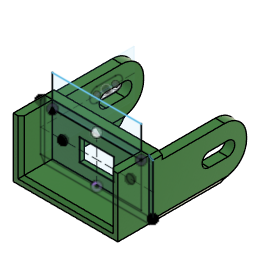
Sensorhalter v8 (Autodesk Fusion 360 design; units mm, degrees)
Autodesk Fusion 360 part; units mm, degrees
sketch "Skizze1" plane through (0, 0, 0) normal (0, 0, 1) x (1, 0, 0)
  line L0 (-18, 30) -> (-18, 0)
  line L1 (-18, 0) -> (18, 0)
  line L2 (18, 0) -> (18, 30)
  line L3 (18, 30) -> (15, 30)
  line L4 (15, 30) -> (15, 3)
  line L5 (15, 3) -> (-15, 3)
  line L6 (-15, 3) -> (-15, 30)
  line L7 (-15, 30) -> (-18, 30)
  line L8 (0, 75) -> (0, -25) construction
  dimension "d1" = 3
  dimension "d2" = 3
  dimension "d3" = 36
  dimension "d4" = 30
  constraint vertical L0
  constraint perpendicular L0 L1
  constraint perpendicular L1 L2
  constraint perpendicular L2 L3
  constraint perpendicular L3 L4
  constraint perpendicular L4 L5
  constraint perpendicular L5 L6
  constraint perpendicular L0 L7
  constraint perpendicular L1 L8
  constraint symmetric L0 L2 L8
  constraint equal L0 L2
  measures "d1" distance of L6.end L0.start
  measures "d2" distance of L1 L5
  measures "d3" distance of L0 L2
  measures "d4" distance of L1 L7
extrude "Extrusion1" add sketch "Skizze1" along normal blind 15
sketch "Skizze2" plane through (-18, 0, 0) normal (-1, 0, 0) x (0, -1, 0)
  line L0 (-30, 0) -> (0, 0)
  line L1 (0, 0) -> (0, 15)
  line L2 (0, 15) -> (-30, 15)
  line L3 (-30, 15) -> (-30, 0)
  line L4 (-30, 7.5) -> (0, 7.5) construction
  line L5 (-24, 9.75) -> (-18, 9.75)
  line L6 (-18, 5.25) -> (-24, 5.25)
  arc A0 (-24, 9.75) -> (-24, 5.25) centre (-24, 7.5) ccw
  arc A1 (-18, 5.25) -> (-18, 9.75) centre (-18, 7.5) ccw
  dimension "d7" = 4.5
  dimension "d8" = 6
  dimension "d9" = 6
  constraint midpoint L3 L4.start
  constraint midpoint L1 L4.end
  constraint coincident L4 A0.centre
  constraint coincident L4 A1.centre
  constraint equal A0 A1
  constraint tangent L5 A0
  constraint tangent L5 A1
  constraint tangent L6 A1
  constraint tangent L6 A0
  measures "d7" diameter of A0
  measures "d8" distance of L3 A0.centre
  measures "d9" distance of A0.centre A1.centre
extrude "Extrusion2" cut sketch "Skizze2" against normal up to surface (36 mm away) contours L5 L6 A0 A1
fillet "Abrundung1" radius 7 4 edges at (-16.5, 30, 15) (16.5, 30, 15) (16.5, 30, 0) (-16.5, 30, 0)
sketch "Skizze3" plane through (0, 0, 0) normal (0, -1, 0) x (1, 0, 0)
  line L0 (-18, 0) -> (18, 0)
  line L1 (18, 0) -> (18, 15)
  line L2 (18, 15) -> (-18, 15)
  line L3 (-18, 15) -> (-18, 0)
  line L4 (18, 7.5) -> (-18, 7.5) construction
  circle A0 centre (10.8, 7.5) radius 1.25
  circle A1 centre (-10.8, 7.5) radius 1.25
  line L5 (14.25, 0.5) -> (-14.25, 0.5)
  line L6 (-14.25, 0.5) -> (-14.25, 14.5)
  line L7 (-14.25, 14.5) -> (14.25, 14.5)
  line L8 (14.25, 14.5) -> (14.25, 0.5)
  line L9 (18, 0) -> (-18, 0)
  line L10 (-18, 0) -> (-18, 15)
  line L11 (18, 16.3062) -> (18, 0)
  line L12 (0, 0) -> (0, 15) construction
  line L13 (16.75, -2) -> (-16.75, -2)
  line L14 (-16.75, -2) -> (-16.75, 17)
  line L15 (-16.75, 17) -> (16.75, 17)
  line L16 (16.75, 17) -> (16.75, -2)
  line L17 (18, 0) -> (16.75, -2)
  line L18 (-18, 0) -> (-16.75, -2)
  line L19 (-18, 15) -> (-16.75, 17)
  line L20 (16.75, 17) -> (18, 16.3062)
  line L21 (-5.5, 4) -> (5.5, 4)
  line L22 (5.5, 4) -> (5.5, 11)
  line L23 (5.5, 11) -> (-5.5, 11)
  line L24 (-5.5, 11) -> (-5.5, 4)
  dimension "d14" = 2.5
  dimension "d15" = 21.6
  dimension "d16" = 14
  dimension "d17" = 28.5
  dimension "d18" = 2.5
  dimension "d19" = 2.5
  dimension "d20" = 2.5
  dimension "d21" = 2.5
  dimension "d28" = 11
  dimension "d29" = 7
  constraint midpoint L1 L4.start
  constraint midpoint L3 L4.end
  constraint coincident L4 A0.centre
  constraint coincident L4 A1.centre
  constraint horizontal L5
  constraint vertical L6
  constraint horizontal L7
  constraint vertical L8
  constraint horizontal L9
  constraint vertical L10
  constraint vertical L11
  constraint coincident L2.end L3.start
  constraint coincident L0.end L1.start
  constraint equal A0 A1
  constraint coincident L12.start origin
  constraint symmetric A0.centre A1.centre L12
  constraint symmetric L4 L5 L7
  constraint symmetric L6 L8 L12
  constraint horizontal L13
  constraint vertical L14
  constraint horizontal L15
  constraint vertical L16
  constraint horizontal L21
  constraint vertical L22
  constraint horizontal L23
  constraint vertical L24
  constraint symmetric L12 L22 L24
  constraint symmetric L4 L21 L23
  measures "d14" diameter of A0
  measures "d15" distance of A0.centre A1.centre
  measures "d16" distance of L5.end L6.end
  measures "d17" distance of L5.start L5.end
  measures "d18" distance of L8 L16
  measures "d19" distance of L6 L14
  measures "d20" distance of L7 L15
  measures "d21" distance of L5 L13
  measures "d28" distance of L21.start L21.end
  measures "d29" distance of L21.end L22.end
extrude "Extrusion3" add sketch "Skizze3" against normal up to surface (3 mm away) contours L0 L9 L14 L18 | L0 L9 L13 L14 L16 | L2 L14 L19 | L0 L9 L16 L17 | L2 L14 L15 L16 | L2 L11 L16 L20
extrude "Extrusion4" cut sketch "Skizze3" against normal up to surface (3 mm away) contours A0 | A1
extrude "Extrusion5" cut sketch "Skizze3" against normal up to surface (3 mm away) contours L21 L22 L23 L24
chamfer "Fase2" distance 1.5 angle 45 4 edges at (0, 3, 4) (5.5, 3, 7.5) (0, 3, 11) (-5.5, 3, 7.5) measured on face at (-1.8333, 3, 15) measured on face at (-1.8333, 3, 15) measured on face at (-1.8333, 3, 15) measured on face at (-1.8333, 3, 15)
extrude "Extrusion6" add sketch "Skizze3" along normal blind 10 contours L0 L2 L9 L14 L16 | L0 L9 L13 L14 L16 | L2 L14 L15 L16
sketch "Skizze5" plane through (0, 0, 7.5) normal (0, -1, 0) x (1, 0, 0)
  line L0 (14.25, 7) -> (-14.25, 7)
  line L1 (-14.25, 7) -> (-14.25, 17)
  line L2 (-14.25, 17) -> (14.25, 17)
  line L3 (14.25, 17) -> (14.25, 7)
  point P0 (-14.25, 7)
  point P1 (14.25, 7)
  constraint horizontal L0
  constraint vertical L1
  constraint horizontal L2
  constraint vertical L3
  constraint coincident P0 L0.end
  constraint coincident L0.start L3.end
extrude "Extrusion8" cut sketch "Skizze5" along normal up to surface (10 mm away)
chamfer "Fase3" distance 1 angle 45 3 edges at (-14.25, -10, 8.75) (0, -10, 0.5) (14.25, -10, 8.75) measured on face at (-4.75, -10, -1.1667) measured on face at (-4.75, -10, -1.1667) measured on face at (-4.75, -10, -1.1667)
sketch "Skizze6" plane through (-18, 15, 7.5) normal (-1, 0, 0) x (0, -1, 0)
  line L0 (-9, 0) -> (-3, 0)
  point P0 (-6, 0)
  constraint horizontal L0
  constraint midpoint L0 P0
sketch "Skizze7" plane through (0, 3, 0) normal (0, 1, 0) x (-1, 0, 0)
  line L0 (15, 0) -> (15, 15)
  line L1 (15, 15) -> (18, 15)
  line L2 (18, 15) -> (16.75, 17)
  line L3 (16.75, 17) -> (-16.75, 17)
  line L4 (-16.75, 17) -> (-18, 16.3062)
  line L5 (-18, 16.3062) -> (-18, 15)
  line L6 (-18, 15) -> (-15, 15)
  line L7 (-15, 15) -> (-15, 0)
  line L8 (-15, 0) -> (-18, 0)
  line L9 (-18, 0) -> (-16.75, -2)
  line L10 (-16.75, -2) -> (16.75, -2)
  line L11 (16.75, -2) -> (18, 0)
  line L12 (18, 0) -> (15, 0)
  circle A0 centre (-10.8, 7.5) radius 1.25
  circle A1 centre (10.8, 7.5) radius 1.25
  line L13 (-7, 12.5) -> (7, 12.5)
  line L14 (7, 12.5) -> (7, 2.5)
  line L15 (7, 2.5) -> (-7, 2.5)
  line L16 (-7, 2.5) -> (-7, 12.5)
  line L17 (15, 0) -> (18, 0)
  line L18 (16.75, -2) -> (15, -2)
  line L19 (15, 0) -> (15, -2)
  line L20 (-15, 0) -> (-15, -2)
  line L21 (-16.75, -2) -> (-18, 0)
  constraint coincident L0.start L12.end
  constraint coincident L11.end L12.start
  constraint coincident L10.end L11.start
  constraint coincident L10 L18.end
  constraint parallel L10 L18
  constraint coincident L7.end L8.start
  constraint coincident L10 L20.end
  constraint perpendicular L10 L20
  constraint coincident L9.end L10.start
  constraint parallel L9 L21
extrude "Extrusion9" add sketch "Skizze7" along normal blind 20 contours L10 L11 L12 L17 L18 L19 | L8 L9 L10 L20 L21
fillet "Abrundung2" radius 2 3 edges at (-15.875, 23, -2) (16.5, 23, 0) (-16.5, 23, 0)
